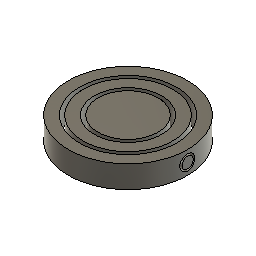
better gyroscope v2 (Autodesk Fusion 360 design; units mm, degrees)
Autodesk Fusion 360 part; units mm, degrees
sketch "Sketch1" plane through (0, 0, 0) normal (0, 1, 0) x (1, 0, 0)
  circle A0 centre (0, 0) radius 8
  circle A1 centre (0, 0) radius 9
  circle A2 centre (0, 0) radius 12
  circle A3 centre (0, 0) radius 13
  circle A4 centre (0, 0) radius 16
  dimension "d4" = 16
  dimension "d5" = 1
  dimension "d6" = 3
  dimension "d7" = 1
  dimension "d8" = 3
  constraint coincident A0.centre A1.centre
  constraint concentric A0 A1
  constraint concentric A1 A2
  constraint concentric A1 A3
  measures "d4" diameter of A0
  measures "d5" distance of A0 A1
  measures "d6" distance of A1 A2
  measures "d7" distance of A2 A3
  measures "d8" distance of A3 A4
extrude "Extrude1" add sketch "Sketch1" along normal mid plane 6 makes body 1 at (1.6626, 3, 1.29) makes body 2 at (11.9851, 2, 0.5982) makes body 3 at (15.9801, 2, 0.7975)
sketch "Sketch2" plane through (0, 0, 0) normal (0, 0, 1) x (1, 0, 0)
  circle A0 centre (0, 0) radius 1.5
  circle A1 centre (0, 0) radius 2
  dimension "d13" = 3
  dimension "d14" = 0.5
  constraint coincident A0.centre A1.centre
  constraint concentric A0 A1
  measures "d13" diameter of A0
  measures "d14" distance of A0 A1
extrude "Extrude2" add sketch "Sketch2" along normal mid plane 24 contours A0 bodies 1
extrude "Extrude3" cut sketch "Sketch2" along normal mid plane 24 contours A0 | A1 bodies 2
sketch "Sketch3" plane through (0, 0, 0) normal (1, 0, 0) x (0, 0, -1)
  circle A0 centre (0, 0) radius 1.5
  circle A1 centre (0, 0) radius 2
  dimension "d19" = 3
  dimension "d20" = 0.5
  constraint coincident A0.centre A1.centre
  constraint concentric A0 A1
  measures "d19" diameter of A0
  measures "d20" distance of A0 A1
extrude "Extrude4" add sketch "Sketch3" along normal blind 7 from surface at 9 contours A0 bodies 2
extrude "Extrude5" add sketch "Sketch3" against normal blind 7 from surface at -9 contours A0 bodies 2
extrude "Extrude6" cut sketch "Sketch3" along normal through all and the other way through all contours A0 | A1 bodies 3
sketch "Sketch4" plane through (0, -3, 0) normal (0, -1, 0) x (1, 0, 0)
  circle A0 centre (0, 0) radius 8
  arc A1 (-2.2094, 1.9868) -> (-5.1841, 2.0472) centre (-3.6929, 2.209) ccw
  line L0 (0, 0) -> (0, 8) construction
  arc A2 (5.1841, 2.0472) -> (2.2094, 1.9868) centre (3.6929, 2.209) ccw
  arc A3 (-4.9, -1.6724) -> (4.9, -1.6724) centre (0, -0.6772) ccw
  arc A4 (-4.9, -1.6724) -> (4.9, -1.6724) centre (0, 9.5513) ccw
  arc A5 (-2.2094, 1.9868) -> (-5.1841, 2.0472) centre (-3.8119, -3.6487) ccw
  arc A6 (5.1841, 2.0472) -> (2.2094, 1.9868) centre (3.8119, -3.6487) ccw
  dimension "d28" = 1.5
  dimension "d29" = 5
  constraint coincident A0.centre L0.start
  constraint coincident A0 L0.end
  constraint vertical L0
  constraint symmetric A1.start L0 A2.end
  constraint symmetric A1.end L0 A2.start
  constraint symmetric A1 L0 A2
  constraint symmetric L0 A3.start A3.end
  constraint coincident A1.centre A5
  constraint symmetric L0 A5 A6
  measures "d28" radius of A1
  measures "d29" radius of A3
extrude "Extrude7" cut sketch "Sketch4" against normal blind 2 contours A1 A5 | A2 A6 | A3 A4 bodies 1
equation "center = 16 mm"
equation "ringspace = 1 mm"
equation "ringwidth = 3 mm"
equation "d4 = center"
equation "d5 = ringspace"
equation "d6 = ringwidth"
equation "d7 = ringspace"
equation "d8 = ringwidth"
equation "rod = 3 mm"
equation "rodspace = 0.5 mm"
equation "d13 = rod"
equation "d14 = rodspace"
equation "d15 = center / 2 + ringspace + ringwidth"
equation "d17 = center / 2 + ringspace + ringwidth"
equation "d19 = rod"
equation "d20 = rodspace"
equation "d21 = center / 2 + ringspace"
equation "d22 = ringwidth + ringspace + ringwidth"
equation "d24 = -center / 2 - ringspace"
equation "d25 = -ringwidth - ringspace - ringwidth"
